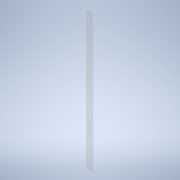
# Autodesk Inventor part: TuerHalter
Saved by Autodesk Inventor 2022 (Build 260153000, 153)
## iProperties
Created: 2021-06-13
Part Number: TuerHalter
Material: Polycarbonate, Clear
Document SubType Name: Modeling
Designer: Cornee
Density: 1.2 g/cm^3
Appearance: Polycarbonate - Clear
Author: Cornee
Autodesk Inventor part; units mm, degrees
ref_plane "YZ Plane" through (0, 0, 0) normal (1, 0, 0) x (0, 1, 0)
ref_plane "XZ Plane" through (0, 0, 0) normal (0, 1, 0) x (-1, 0, 0)
ref_plane "XY Plane" through (0, 0, 0) normal (0, 0, 1) x (1, 0, 0)
sketch "Sketch1" plane through (0, 0, 0) normal (0, 0, 1) x (1, 0, 0)
  line L0 (-33.8284, 8.2949) -> (2.1716, 8.2949)
  line L1 (2.1716, 8.2949) -> (2.1716, 713.2949)
  line L2 (2.1716, 713.2949) -> (-33.8284, 713.2949)
  line L3 (-33.8284, 713.2949) -> (-33.8284, 8.2949)
  circle A0 centre (-19.8284, 670.7949) radius 3
  circle A1 centre (-19.8284, 650.7949) radius 3
  circle A2 centre (-19.8284, 70.7949) radius 3
  circle A3 centre (-19.8284, 50.7949) radius 3
  circle A4 centre (-19.8284, 370.7949) radius 3
  circle A5 centre (-19.8284, 350.7949) radius 3
  circle A6 centre (-5.8284, 250.7949) radius 2.25
  circle A7 centre (-5.8284, 30.7949) radius 2.25
  circle A8 centre (-5.8284, 690.7949) radius 2.25
  circle A9 centre (-5.8284, 470.7949) radius 2
  point P0 (0, 0)
  dimension "d0" = 36
  dimension "d1" = 705
  dimension "d2" = 6
  dimension "d3" = 6
  dimension "d4" = 20
  dimension "d5" = 6
  dimension "d6" = 6
  dimension "d7" = 20
  dimension "d8" = 600
  dimension "d9" = 42.5
  dimension "d10" = 14
  dimension "d13" = 6
  dimension "d14" = 6
  dimension "d15" = 20
  dimension "d16" = 300
  dimension "d21" = 4.5
  dimension "d22" = 4.5
  dimension "d23" = 4.5
  dimension "d24" = 4
  dimension "d25" = 8
  dimension "d26" = 220
  dimension "d27" = 220
  dimension "d28" = 220
  dimension "d29" = 22.5
  constraints: 10 centre point, 8 end point, 8 vertical alignment, 2 parallel, 1 horizontal, 1 perpendicular
  measures "d0" distance of L2.end L1.end
  measures "d1" distance of L1.end L0.end
  measures "d2" diameter of A0
  measures "d3" diameter of A1
  measures "d4" distance of A1.centre A0.centre
  measures "d5" diameter of A2
  measures "d6" diameter of A3
  measures "d7" distance of A3.centre A2.centre
  measures "d8" distance of A2.centre A0.centre
  measures "d9" distance from line of L0 A3.centre
  measures "d10" distance from line of L3 A3.centre
  measures "d13" diameter of A4
  measures "d14" diameter of A5
  measures "d15" distance of A5.centre A4.centre
  measures "d16" distance of A4.centre A2.centre
  measures "d21" diameter of A6
  measures "d22" diameter of A7
  measures "d23" diameter of A8
  measures "d24" diameter of A9
  measures "d25" distance from line of L1 A7.centre
  measures "d26" distance of A6.centre A7.centre
  measures "d27" distance of A6.centre A9.centre
  measures "d28" distance of A9.centre A8.centre
  measures "d29" distance from line of L0 A7.centre
extrude "Extrusion1" add sketch "Sketch1" along normal blind 5 contours L3 L2 L1 L0 | A4 | A5 | A6 | A7 | A8 | A9
extrude "Extrusion2" cut sketch "Sketch1" along normal blind 3 contours A5
extrude "Extrusion3" cut sketch "Sketch1" along normal blind 3 contours A4
extrude "Extrusion4" cut sketch "Sketch1" along normal blind 3 contours A6 | A7 | A8 | A9
equation "\"d27\" = d26"
equation "\"d28\" = d26"
body "Solid1"
